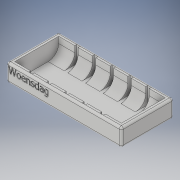
# Autodesk Inventor part: Woendag
Saved by Autodesk Inventor 2019 (Build 230136000, 136)
## iProperties
Created: 2020-10-20
Part Number: Woendag
Material: Generic
Document SubType Name: Modeling
Designer: daanswinters
Density: 1 g/cm^3
Appearance: Default
Author: daanswinters
Autodesk Inventor part; units mm, degrees
ref_plane "YZ Plane" through (0, 0, 0) normal (1, 0, 0) x (0, 1, 0)
ref_plane "XZ Plane" through (0, 0, 0) normal (0, 1, 0) x (-1, 0, 0)
ref_plane "XY Plane" through (0, 0, 0) normal (0, 0, 1) x (1, 0, 0)
sketch "Sketch1" plane through (0, 0, 0) normal (0, 0, 1) x (1, 0, 0)
  line L0 (55, -8.5) -> (-55, -8.5)
  line L1 (-55, -8.5) -> (-55, 8.5)
  line L2 (-55, 8.5) -> (55, 8.5)
  line L3 (55, 8.5) -> (55, -8.5)
  line L4 (55, -8.5) -> (-55, 8.5) construction
  line L5 (-55, -8.5) -> (55, 8.5) construction
  point P0 (0, 0)
  dimension "d0" = 110
  dimension "d1" = 17
  constraints: 12 end point, 2 midpoint, 2 parallel, 1 horizontal, 1 perpendicular
  measures "d0" distance of L1.end L2.end
  measures "d1" distance of L0.end L1.end
extrude "Extrusion1" add sketch "Sketch1" along normal blind 50
sketch "Sketch2" plane through (-55, 8.5, 0) normal (0, 1, 0) x (1, 0, 0)
  line L0 (0, 0) -> (0, -50) projected
  line L1 (110, -50) -> (0, -50)
  line L2 (0, -50) -> (0, 0)
  line L3 (0, 0) -> (110, 0)
  line L4 (110, 0) -> (110, -50)
  line L5 (110, -50) -> (0, 0) construction
  line L6 (0, -50) -> (110, 0) construction
  line L7 (106, -46) -> (106, -4)
  line L8 (4, -4) -> (4, -46)
  line L9 (56.15, -2) -> (53.85, -2)
  line L10 (53.85, -48) -> (56.15, -48)
  line L11 (56.15, -2) -> (53.85, -48) construction
  line L12 (53.85, -2) -> (56.15, -48) construction
  line L13 (73.15, -2) -> (70.85, -2)
  line L14 (70.85, -48) -> (73.15, -48)
  line L15 (73.15, -2) -> (70.85, -48) construction
  line L16 (70.85, -2) -> (73.15, -48) construction
  line L17 (0, -25) -> (110, -25) construction
  line L18 (87.85, -2) -> (90.15, -2)
  line L19 (90.15, -48) -> (87.85, -48)
  line L20 (87.85, -2) -> (90.15, -48) construction
  line L21 (90.15, -2) -> (87.85, -48) construction
  line L22 (36.85, -2) -> (39.15, -2)
  line L23 (39.15, -48) -> (36.85, -48)
  line L24 (36.85, -2) -> (39.15, -48) construction
  line L25 (39.15, -2) -> (36.85, -48) construction
  line L26 (19.85, -2) -> (22.15, -2)
  line L27 (22.15, -48) -> (19.85, -48)
  line L28 (19.85, -2) -> (22.15, -48) construction
  line L29 (22.15, -2) -> (19.85, -48) construction
  line L30 (90.15, -2) -> (90.15, -4)
  line L31 (90.15, -46) -> (90.15, -48)
  line L32 (87.85, -48) -> (87.85, -46)
  line L33 (87.85, -4) -> (87.85, -2)
  line L34 (73.15, -48) -> (73.15, -46)
  line L35 (73.15, -4) -> (73.15, -2)
  line L36 (70.85, -2) -> (70.85, -4)
  line L37 (70.85, -46) -> (70.85, -48)
  line L38 (56.15, -4) -> (56.15, -2)
  line L39 (53.85, -2) -> (53.85, -4)
  line L40 (53.85, -46) -> (53.85, -48)
  line L41 (56.15, -48) -> (56.15, -46)
  line L42 (39.15, -2) -> (39.15, -4)
  line L43 (39.15, -46) -> (39.15, -48)
  line L44 (36.85, -48) -> (36.85, -46)
  line L45 (36.85, -4) -> (36.85, -2)
  line L46 (22.15, -2) -> (22.15, -4)
  line L47 (19.85, -48) -> (19.85, -46)
  line L48 (19.85, -4) -> (19.85, -2)
  line L49 (22.15, -46) -> (22.15, -48)
  line L50 (4, -46) -> (19.95, -46)
  line L51 (22.05, -46) -> (36.95, -46)
  line L52 (39.05, -46) -> (53.95, -46)
  line L53 (56.05, -46) -> (70.95, -46)
  line L54 (73.05, -46) -> (87.95, -46)
  line L55 (90.05, -46) -> (106, -46)
  line L56 (106, -4) -> (90.05, -4)
  line L57 (87.95, -4) -> (73.05, -4)
  line L58 (70.95, -4) -> (56.05, -4)
  line L59 (53.95, -4) -> (39.05, -4)
  line L60 (36.95, -4) -> (22.05, -4)
  line L61 (19.95, -4) -> (4, -4)
  point P0 (55, 0)
  point P1 (55, -25)
  point P2 (72, -25)
  point P3 (89, -25)
  point P4 (38, -25)
  point P5 (21, -25)
  dimension "d4" = 65.556
  dimension "d5" = 110
  dimension "d7" = 2.3
  dimension "d8" = 46
  dimension "d9" = 2.3
  dimension "d10" = 46
  dimension "d11" = 0
  dimension "d12" = 2.3
  dimension "d13" = 46
  dimension "d14" = 2.3
  dimension "d15" = 46
  dimension "d16" = 2.3
  dimension "d17" = 46
  dimension "d18" = 17
  dimension "d19" = 17
  dimension "d20" = 17
  dimension "d21" = 17
  dimension "d22" = 2.862
  dimension "d23" = 2.862
  dimension "d24" = 106
  dimension "d25" = 4
  dimension "d26" = 42
  dimension "d27" = 2
  dimension "d28" = 0
  dimension "d29" = 42
  dimension "d30" = 0
  dimension "d31" = 42
  dimension "d32" = 0
  dimension "d33" = 42
  dimension "d34" = 0
  dimension "d35" = 42
  dimension "d36" = 0
  dimension "d37" = 42
  constraints: 122 end point, 73 parallel, 43 point on line, 17 perpendicular, 14 midpoint, 6 horizontal
  measures "d4" angle of L5 L0
  measures "d5" distance between parallel lines of L4 L0
  measures "d7" distance of L10.end L10.start
  measures "d8" distance of L10.start L9.end
  measures "d9" distance of L14.end L14.start
  measures "d10" distance of L14.start L13.end
  measures "d11" distance from line of L17 point (72, -25)
  measures "d12" distance of L19.start L19.end
  measures "d13" distance of L18.end L19.start
  measures "d14" distance of L23.start L23.end
  measures "d15" distance of L22.end L23.start
  measures "d16" distance of L27.start L27.end
  measures "d17" distance of L26.end L27.start
  measures "d18" distance of point (72, -25) point (55, -25)
  measures "d19" distance of point (89, -25) point (72, -25)
  measures "d20" distance of point (38, -25) point (55, -25)
  measures "d21" distance of point (21, -25) point (38, -25)
  measures "d22" angle of L0 L20
  measures "d23" angle of L0 L21
  measures "d24" distance between parallel lines of L7 L0
  measures "d25" distance between parallel lines of L8 L0
  measures "d26" distance between parallel lines of L56 L55
  measures "d27" distance between parallel lines of L56 L18
  measures "d28" distance between parallel lines of L56 L57
  measures "d29" distance between parallel lines of L56 L54
  measures "d30" distance between parallel lines of L56 L58
  measures "d31" distance between parallel lines of L56 L53
  measures "d32" distance between parallel lines of L56 L59
  measures "d33" distance between parallel lines of L56 L52
  measures "d34" distance between parallel lines of L56 L60
  measures "d35" distance between parallel lines of L56 L51
  measures "d36" distance between parallel lines of L56 L61
  measures "d37" distance between parallel lines of L56 L50
extrude "Extrusion2" cut sketch "Sketch2" against normal blind 16 contours L55 L31 L19 L32 L54 L34 L14 L37 L53 L41 L10 L40 L52 L43 L23 L44 L51 L49 L27 L47 L50 L8 L61 L48 L26 L46 L60 L45 L22 L42 L59 L39 L9 L38 L58 L36 L13 L35 L57 L33 L18 L30 L56 L7
fillet "Fillet1" radius 2 12 edges at (-55, 0, 50) (-55, 0, 0) (55, 0, 50) (55, 0, 0) (0, 8.5, 50) (-55, 8.5, 25) (0, 8.5, 0) (55, 8.5, 25) (55, -8.5, 25) (0, -8.5, 50) (-55, -8.5, 25) (0, -8.5, 0)
fillet "Fillet2" radius 10 6 edges at (-43.075, -7.5, 4) (-25.5, -7.5, 4) (-8.5, -7.5, 4) (8.5, -7.5, 4) (25.5, -7.5, 4) (43.075, -7.5, 4)
sketch "Sketch3" plane through (35.15, 8.5, 4) normal (0, 1, 0) x (1, 0, 0)
  line L0 (-70.3, -44) -> (-70.3, -42) projected
  line L1 (-51, 2) -> (-53.3, 2)
  line L2 (-34, 2) -> (-34, 0) projected
  line L3 (-36.3, -44) -> (-36.3, -42) projected
  line L4 (-19.3, -44) -> (-19.3, -42) projected
  line L5 (-2.3, -44) -> (-2.3, -42) projected
  line L6 (0, 2) -> (0, 0) projected
  line L7 (-19.8, 2) -> (-16.5, 2)
  line L8 (-16.5, 2) -> (-16.5, -44)
  line L9 (-16.5, -44) -> (-19.8, -44)
  line L10 (-19.8, -44) -> (-19.8, 2)
  line L11 (-19.8, 2) -> (-16.5, -44) construction
  line L12 (-16.5, 2) -> (-19.8, -44) construction
  line L13 (-2.8, -44) -> (0.5, -44)
  line L14 (0.5, -44) -> (0.5, 2)
  line L15 (0.5, 2) -> (-2.8, 2)
  line L16 (-2.8, 2) -> (-2.8, -44)
  line L17 (-2.8, -44) -> (0.5, 2) construction
  line L18 (0.5, -44) -> (-2.8, 2) construction
  line L19 (-36.8, -44) -> (-33.5, -44)
  line L20 (-33.5, -44) -> (-33.5, 2)
  line L21 (-33.5, 2) -> (-36.8, 2)
  line L22 (-36.8, 2) -> (-36.8, -44)
  line L23 (-36.8, -44) -> (-33.5, 2) construction
  line L24 (-33.5, -44) -> (-36.8, 2) construction
  line L25 (-51, 2) -> (-36.3, 2) projected
  line L26 (-53.8, -44) -> (-50.5, -44)
  line L27 (-50.5, -44) -> (-50.5, 2)
  line L28 (-50.5, 2) -> (-53.8, 2)
  line L29 (-53.8, 2) -> (-53.8, -44)
  line L30 (-53.8, -44) -> (-50.5, 2) construction
  line L31 (-50.5, -44) -> (-53.8, 2) construction
  line L32 (-53.3, -44) -> (-68, -44) projected
  line L33 (-70.8, 2) -> (-67.5, 2)
  line L34 (-67.5, 2) -> (-67.5, -44)
  line L35 (-67.5, -44) -> (-70.8, -44)
  line L36 (-70.8, -44) -> (-70.8, 2)
  line L37 (-70.8, 2) -> (-67.5, -44) construction
  line L38 (-67.5, 2) -> (-70.8, -44) construction
  point P0 (-35.15, 4)
  point P1 (-68, 2)
  point P2 (-17, 2)
  point P3 (-18.15, -21)
  point P4 (-1.15, -21)
  point P5 (-35.15, -21)
  point P6 (-52.15, -21)
  point P7 (-69.15, -21)
  dimension "d42" = 3.3
  dimension "d43" = 46
  dimension "d44" = 3.3
  dimension "d45" = 3.3
  dimension "d46" = 3.3
  dimension "d47" = 3.3
  dimension "d48" = 90
  dimension "d49" = 0.5
  dimension "d50" = 16.5
  dimension "d51" = 33.5
  dimension "d52" = 50.5
  dimension "d53" = 67.5
  dimension "d54" = 46
  dimension "d55" = 0
  dimension "d56" = 53.3
  constraints: 62 end point, 14 parallel, 10 midpoint, 5 horizontal, 5 perpendicular, 3 point on line
  measures "d42" distance of L8.end L9.end
  measures "d43" distance of L7.end L8.end
  measures "d44" distance of L15.end L14.end
  measures "d45" distance of L21.end L20.end
  measures "d46" distance of L28.end L27.end
  measures "d47" distance of L34.end L35.end
  measures "d48" angle of L6 L1
  measures "d49" distance between parallel lines of L6 L14
  measures "d50" distance between parallel lines of L6 L8
  measures "d51" distance between parallel lines of L6 L20
  measures "d52" distance between parallel lines of L6 L27
  measures "d53" distance between parallel lines of L6 L34
  measures "d54" distance between parallel lines of L25 L9
  measures "d55" distance between parallel lines of L15 L25
  measures "d56" distance from line of L1.end L6
extrude "Extrusion3" cut sketch "Sketch3" against normal blind 16
sketch "Sketch4" plane through (0, 0, 50) normal (0, 0, 1) x (1, 0, 0)
  line L0 (-52.9749, 6.5012) -> (53.0345, 6.5012) construction
  line L1 (53.0345, 6.5012) -> (53.0345, -6.5247) construction
  line L2 (53.0345, -6.5247) -> (-52.9749, -6.5247) construction
  line L3 (-52.9749, -6.5247) -> (-52.9749, 6.5012) construction
  line L4 (-45.5205, 6.2294) -> (-47.0529, 0.1294)
  line L5 (-47.0529, 0.1294) -> (-47.9624, 0.1294)
  line L6 (-47.9624, 0.1294) -> (-49.2032, 5.1913)
  line L7 (-49.2032, 5.1913) -> (-50.4094, 0.1294)
  line L8 (-50.4094, 0.1294) -> (-51.309, 0.1294)
  line L9 (-51.309, 0.1294) -> (-52.8662, 6.2294)
  line L10 (-52.8662, 6.2294) -> (-52.0308, 6.2294)
  line L11 (-52.0308, 6.2294) -> (-50.8048, 1.1724)
  line L12 (-50.8048, 1.1724) -> (-49.5888, 6.2294)
  line L13 (-49.5888, 6.2294) -> (-48.7633, 6.2294)
  line L14 (-48.7633, 6.2294) -> (-47.5373, 1.1131)
  line L15 (-47.5373, 1.1131) -> (-46.3163, 6.2294)
  line L16 (-46.3163, 6.2294) -> (-45.5205, 6.2294)
  spline S0 degree 2 poles (-41.0913, 2.4181) (-41.0913, 1.2614) (-42.2035, 0.0008) (-43.1329, 0.0008) knots 0 0 0 1 2 2 2
  spline S1 degree 2 poles (-43.1329, 0.0008) (-44.0869, 0.0008) (-45.1794, 1.3009) (-45.1794, 2.4181) knots 0 0 0 1 2 2 2
  spline S2 degree 2 poles (-45.1794, 2.4181) (-45.1794, 3.5649) (-44.0523, 4.8354) (-43.1329, 4.8354) knots 0 0 0 1 2 2 2
  spline S3 degree 2 poles (-43.1329, 4.8354) (-42.2035, 4.8354) (-41.0913, 3.5699) (-41.0913, 2.4181) knots 0 0 0 1 2 2 2
  spline S4 degree 2 poles (-41.8872, 2.4181) (-41.8872, 3.3079) (-42.5347, 4.173) (-43.1329, 4.173) knots 0 0 0 1 2 2 2
  spline S5 degree 2 poles (-43.1329, 4.173) (-43.731, 4.173) (-44.3835, 3.3079) (-44.3835, 2.4181) knots 0 0 0 1 2 2 2
  spline S6 degree 2 poles (-44.3835, 2.4181) (-44.3835, 1.553) (-43.731, 0.6632) (-43.1329, 0.6632) knots 0 0 0 1 2 2 2
  spline S7 degree 2 poles (-43.1329, 0.6632) (-42.5397, 0.6632) (-41.8872, 1.5382) (-41.8872, 2.4181) knots 0 0 0 1 2 2 2
  spline S8 degree 2 poles (-38.3132, 0.0256) (-39.4106, 0.0256) (-40.6167, 1.2564) (-40.6167, 2.3934) knots 0 0 0 1 2 2 2
  spline S9 degree 2 poles (-40.6167, 2.3934) (-40.6167, 3.5106) (-39.4452, 4.8354) (-38.501, 4.8354) knots 0 0 0 1 2 2 2
  spline S10 degree 2 poles (-38.501, 4.8354) (-38.0759, 4.8354) (-37.4184, 4.5882) (-37.1762, 4.3262) knots 0 0 0 1 2 2 2
  spline S11 degree 2 poles (-37.1762, 4.3262) (-36.9291, 4.0642) (-36.6671, 3.3079) (-36.6671, 2.7592) knots 0 0 0 1 2 2 2
  line L17 (-36.6671, 2.7592) -> (-36.6671, 2.339)
  line L18 (-36.6671, 2.339) -> (-39.8357, 2.339)
  spline S12 degree 2 poles (-39.8357, 2.339) (-39.8357, 1.5431) (-39.0349, 0.6978) (-38.3231, 0.6978) knots 0 0 0 1 2 2 2
  spline S13 degree 2 poles (-38.3231, 0.6978) (-38.071, 0.6978) (-37.5816, 0.8115) (-37.3838, 0.9005) knots 0 0 0 1 2 2 2
  spline S14 degree 2 poles (-37.3838, 0.9005) (-37.1762, 0.9994) (-36.8895, 1.1724) (-36.7956, 1.2515) knots 0 0 0 1 2 2 2
  line L19 (-36.7956, 1.2515) -> (-36.7511, 1.2515)
  line L20 (-36.7511, 1.2515) -> (-36.7511, 0.4111)
  spline S15 degree 2 poles (-36.7511, 0.4111) (-36.8846, 0.3568) (-37.2899, 0.1986) (-37.4481, 0.1541) knots 0 0 0 1 2 2 2
  spline S16 degree 2 poles (-37.4481, 0.1541) (-37.6706, 0.0898) (-38.0364, 0.0256) (-38.3132, 0.0256) knots 0 0 0 1 2 2 2
  spline S17 degree 2 poles (-37.4184, 2.9273) (-37.4283, 3.2387) (-37.5569, 3.6935) (-37.6804, 3.8467) knots 0 0 0 1 2 2 2
  spline S18 degree 2 poles (-37.6804, 3.8467) (-37.8139, 4.0197) (-38.2341, 4.2026) (-38.5455, 4.2026) knots 0 0 0 1 2 2 2
  spline S19 degree 2 poles (-38.5455, 4.2026) (-38.852, 4.2026) (-39.2821, 4.0197) (-39.46, 3.8418) knots 0 0 0 1 2 2 2
  spline S20 degree 2 poles (-39.46, 3.8418) (-39.633, 3.6589) (-39.811, 3.2189) (-39.8357, 2.9273) knots 0 0 0 1 2 2 2
  line L21 (-39.8357, 2.9273) -> (-37.4184, 2.9273)
  line L22 (-32.2923, 0.1294) -> (-33.0634, 0.1294)
  line L23 (-33.0634, 0.1294) -> (-33.0634, 2.7394)
  spline S21 degree 2 poles (-33.0634, 2.7394) (-33.0634, 3.0558) (-33.1227, 3.5995) (-33.2117, 3.7627) knots 0 0 0 1 2 2 2
  spline S22 degree 2 poles (-33.2117, 3.7627) (-33.3056, 3.9357) (-33.6418, 4.1038) (-33.9285, 4.1038) knots 0 0 0 1 2 2 2
  spline S23 degree 2 poles (-33.9285, 4.1038) (-34.2152, 4.1038) (-34.8232, 3.7973) (-35.1149, 3.5501) knots 0 0 0 1 2 2 2
  line L24 (-35.1149, 3.5501) -> (-35.1149, 0.1294)
  line L25 (-35.1149, 0.1294) -> (-35.886, 0.1294)
  line L26 (-35.886, 0.1294) -> (-35.886, 4.7068)
  line L27 (-35.886, 4.7068) -> (-35.1149, 4.7068)
  line L28 (-35.1149, 4.7068) -> (-35.1149, 4.1977)
  spline S24 degree 2 poles (-35.1149, 4.1977) (-34.7688, 4.5091) (-34.1015, 4.8354) (-33.7258, 4.8354) knots 0 0 0 1 2 2 2
  spline S25 degree 2 poles (-33.7258, 4.8354) (-33.0535, 4.8354) (-32.2923, 3.9456) (-32.2923, 3.1003) knots 0 0 0 1 2 2 2
  line L29 (-32.2923, 3.1003) -> (-32.2923, 0.1294)
  spline S26 degree 2 poles (-29.9739, 0.0206) (-30.4336, 0.0206) (-31.2295, 0.2678) (-31.4915, 0.4062) knots 0 0 0 1 2 2 2
  line L30 (-31.4915, 0.4062) -> (-31.4915, 1.2713)
  line L31 (-31.4915, 1.2713) -> (-31.4519, 1.2713)
  spline S27 degree 2 poles (-31.4519, 1.2713) (-31.353, 1.1922) (-31.0861, 1.0043) (-30.8637, 0.9005) knots 0 0 0 1 2 2 2
  spline S28 degree 2 poles (-30.8637, 0.9005) (-30.6709, 0.8066) (-30.1963, 0.6682) (-29.9442, 0.6682) knots 0 0 0 1 2 2 2
  spline S29 degree 2 poles (-29.9442, 0.6682) (-29.7613, 0.6682) (-29.3411, 0.7522) (-29.2423, 0.8214) knots 0 0 0 1 2 2 2
  spline S30 degree 2 poles (-29.2423, 0.8214) (-29.0989, 0.9153) (-28.9704, 1.1279) (-28.9704, 1.3454) knots 0 0 0 1 2 2 2
  spline S31 degree 2 poles (-28.9704, 1.3454) (-28.9704, 1.6173) (-29.267, 1.8991) (-29.6476, 1.993) knots 0 0 0 1 2 2 2
  spline S32 degree 2 poles (-29.6476, 1.993) (-29.7959, 2.0276) (-30.2705, 2.1265) (-30.4731, 2.1808) knots 0 0 0 1 2 2 2
  spline S33 degree 2 poles (-30.4731, 2.1808) (-30.9971, 2.3341) (-31.4717, 2.9668) (-31.4717, 3.4166) knots 0 0 0 1 2 2 2
  spline S34 degree 2 poles (-31.4717, 3.4166) (-31.4717, 4.0395) (-30.5374, 4.8156) (-29.7663, 4.8156) knots 0 0 0 1 2 2 2
  spline S35 degree 2 poles (-29.7663, 4.8156) (-29.3856, 4.8156) (-28.6145, 4.6277) (-28.3525, 4.4844) knots 0 0 0 1 2 2 2
  line L32 (-28.3525, 4.4844) -> (-28.3525, 3.6589)
  line L33 (-28.3525, 3.6589) -> (-28.392, 3.6589)
  spline S36 degree 2 poles (-28.392, 3.6589) (-28.6886, 3.8961) (-29.4103, 4.168) (-29.7811, 4.168) knots 0 0 0 1 2 2 2
  spline S37 degree 2 poles (-29.7811, 4.168) (-30.1617, 4.168) (-30.6857, 3.8467) (-30.6857, 3.5254) knots 0 0 0 1 2 2 2
  spline S38 degree 2 poles (-30.6857, 3.5254) (-30.6857, 3.2337) (-30.3743, 2.952) (-30.0282, 2.863) knots 0 0 0 1 2 2 2
  spline S39 degree 2 poles (-30.0282, 2.863) (-29.8602, 2.8185) (-29.4351, 2.7295) (-29.2027, 2.6752) knots 0 0 0 1 2 2 2
  spline S40 degree 2 poles (-29.2027, 2.6752) (-28.6985, 2.5466) (-28.1844, 1.9584) (-28.1844, 1.4492) knots 0 0 0 1 2 2 2
  spline S41 degree 2 poles (-28.1844, 1.4492) (-28.1844, 1.1526) (-28.4167, 0.6286) (-28.6441, 0.4359) knots 0 0 0 1 2 2 2
  spline S42 degree 2 poles (-28.6441, 0.4359) (-28.8864, 0.2332) (-29.5043, 0.0206) (-29.9739, 0.0206) knots 0 0 0 1 2 2 2
  line L34 (-23.948, 0.1294) -> (-24.7192, 0.1294)
  line L35 (-24.7192, 0.1294) -> (-24.7192, 0.594)
  spline S43 degree 2 poles (-24.7192, 0.594) (-24.8971, 0.4457) (-25.1591, 0.248) (-25.3371, 0.164) knots 0 0 0 1 2 2 2
  spline S44 degree 2 poles (-25.3371, 0.164) (-25.5002, 0.0849) (-25.8512, 0.0008) (-26.0835, 0.0008) knots 0 0 0 1 2 2 2
  spline S45 degree 2 poles (-26.0835, 0.0008) (-26.4592, 0.0008) (-27.0919, 0.3123) (-27.3144, 0.6138) knots 0 0 0 1 2 2 2
  spline S46 degree 2 poles (-27.3144, 0.6138) (-27.5368, 0.9153) (-27.784, 1.8051) (-27.784, 2.3835) knots 0 0 0 1 2 2 2
  spline S47 degree 2 poles (-27.784, 2.3835) (-27.784, 2.9866) (-27.4726, 3.8665) (-27.2007, 4.1977) knots 0 0 0 1 2 2 2
  spline S48 degree 2 poles (-27.2007, 4.1977) (-26.9486, 4.4943) (-26.2417, 4.8354) (-25.8512, 4.8354) knots 0 0 0 1 2 2 2
  spline S49 degree 2 poles (-25.8512, 4.8354) (-25.5101, 4.8354) (-25.0009, 4.6821) (-24.7192, 4.5239) knots 0 0 0 1 2 2 2
  line L36 (-24.7192, 4.5239) -> (-24.7192, 6.5012)
  line L37 (-24.7192, 6.5012) -> (-23.948, 6.5012)
  line L38 (-23.948, 6.5012) -> (-23.948, 0.1294)
  line L39 (-24.7192, 1.2416) -> (-24.7192, 3.8863)
  spline S50 degree 2 poles (-24.7192, 3.8863) (-25.0059, 4.0247) (-25.4607, 4.1285) (-25.7227, 4.1285) knots 0 0 0 1 2 2 2
  spline S51 degree 2 poles (-25.7227, 4.1285) (-26.3158, 4.1285) (-26.9881, 3.2387) (-26.9881, 2.3983) knots 0 0 0 1 2 2 2
  spline S52 degree 2 poles (-26.9881, 2.3983) (-26.9881, 1.5876) (-26.474, 0.7324) (-25.9056, 0.7324) knots 0 0 0 1 2 2 2
  spline S53 degree 2 poles (-25.9056, 0.7324) (-25.604, 0.7324) (-24.9911, 1.0093) (-24.7192, 1.2416) knots 0 0 0 1 2 2 2
  spline S54 degree 2 poles (-20.2801, 0.6138) (-20.374, 0.5446) (-20.6904, 0.2974) (-20.8387, 0.2233) knots 0 0 0 1 2 2 2
  spline S55 degree 2 poles (-20.8387, 0.2233) (-21.0414, 0.1145) (-21.422, 0.0008) (-21.768, 0.0008) knots 0 0 0 1 2 2 2
  spline S56 degree 2 poles (-21.768, 0.0008) (-22.0498, 0.0008) (-22.559, 0.2134) (-22.7517, 0.4062) knots 0 0 0 1 2 2 2
  spline S57 degree 2 poles (-22.7517, 0.4062) (-22.9347, 0.594) (-23.1571, 1.1477) (-23.1571, 1.4542) knots 0 0 0 1 2 2 2
  spline S58 degree 2 poles (-23.1571, 1.4542) (-23.1571, 1.9287) (-22.7567, 2.601) (-22.3217, 2.7938) knots 0 0 0 1 2 2 2
  spline S59 degree 2 poles (-22.3217, 2.7938) (-21.9361, 2.9718) (-20.8881, 3.1052) (-20.2801, 3.1398) knots 0 0 0 1 2 2 2
  line L40 (-20.2801, 3.1398) -> (-20.2801, 3.2881)
  spline S60 degree 2 poles (-20.2801, 3.2881) (-20.2801, 3.5551) (-20.4432, 3.8863) (-20.5915, 3.9802) knots 0 0 0 1 2 2 2
  spline S61 degree 2 poles (-20.5915, 3.9802) (-20.7398, 4.0741) (-21.165, 4.1334) (-21.3923, 4.1334) knots 0 0 0 1 2 2 2
  spline S62 degree 2 poles (-21.3923, 4.1334) (-21.6593, 4.1334) (-22.381, 3.9752) (-22.7419, 3.822) knots 0 0 0 1 2 2 2
  line L41 (-22.7419, 3.822) -> (-22.7864, 3.822)
  line L42 (-22.7864, 3.822) -> (-22.7864, 4.608)
  spline S63 degree 2 poles (-22.7864, 4.608) (-22.5738, 4.6673) (-21.7779, 4.8156) (-21.3874, 4.8156) knots 0 0 0 1 2 2 2
  spline S64 degree 2 poles (-21.3874, 4.8156) (-20.9129, 4.8156) (-20.2653, 4.6673) (-20.0082, 4.4745) knots 0 0 0 1 2 2 2
  spline S65 degree 2 poles (-20.0082, 4.4745) (-19.7561, 4.2867) (-19.509, 3.6885) (-19.509, 3.2585) knots 0 0 0 1 2 2 2
  line L43 (-19.509, 3.2585) -> (-19.509, 0.1294)
  line L44 (-19.509, 0.1294) -> (-20.2801, 0.1294)
  line L45 (-20.2801, 0.1294) -> (-20.2801, 0.6138)
  line L46 (-20.2801, 1.2564) -> (-20.2801, 2.5269)
  spline S66 degree 2 poles (-20.2801, 2.5269) (-20.5569, 2.5021) (-21.3923, 2.4181) (-21.6543, 2.339) knots 0 0 0 1 2 2 2
  spline S67 degree 2 poles (-21.6543, 2.339) (-21.9608, 2.2451) (-22.3612, 1.8546) (-22.3612, 1.5085) knots 0 0 0 1 2 2 2
  spline S68 degree 2 poles (-22.3612, 1.5085) (-22.3612, 1.1131) (-21.9163, 0.7127) (-21.4912, 0.7127) knots 0 0 0 1 2 2 2
  spline S69 degree 2 poles (-21.4912, 0.7127) (-21.1304, 0.7127) (-20.5372, 1.0241) (-20.2801, 1.2564) knots 0 0 0 1 2 2 2
  spline S70 degree 2 poles (-18.2633, -0.6022) (-18.1842, -0.6368) (-17.8826, -0.7456) (-17.6898, -0.7901) knots 0 0 0 1 2 2 2
  spline S71 degree 2 poles (-17.6898, -0.7901) (-17.4773, -0.8445) (-17.1164, -0.9087) (-16.9039, -0.9087) knots 0 0 0 1 2 2 2
  spline S72 degree 2 poles (-16.9039, -0.9087) (-16.5479, -0.9087) (-16.0536, -0.7209) (-15.9152, -0.5528) knots 0 0 0 1 2 2 2
  spline S73 degree 2 poles (-15.9152, -0.5528) (-15.7817, -0.3847) (-15.6779, 0.0552) (-15.6779, 0.337) knots 0 0 0 1 2 2 2
  line L47 (-15.6779, 0.337) -> (-15.6779, 0.7374)
  spline S74 degree 2 poles (-15.6779, 0.7374) (-15.9894, 0.4655) (-16.5875, 0.2085) (-17.0373, 0.2085) knots 0 0 0 1 2 2 2
  spline S75 degree 2 poles (-17.0373, 0.2085) (-17.8184, 0.2085) (-18.7428, 1.3701) (-18.7428, 2.4626) knots 0 0 0 1 2 2 2
  spline S76 degree 2 poles (-18.7428, 2.4626) (-18.7428, 3.0311) (-18.4214, 3.911) (-18.1545, 4.2224) knots 0 0 0 1 2 2 2
  spline S77 degree 2 poles (-18.1545, 4.2224) (-17.8975, 4.5141) (-17.1906, 4.8354) (-16.8149, 4.8354) knots 0 0 0 1 2 2 2
  spline S78 degree 2 poles (-16.8149, 4.8354) (-16.459, 4.8354) (-15.9399, 4.6673) (-15.6779, 4.5141) knots 0 0 0 1 2 2 2
  line L48 (-15.6779, 4.5141) -> (-15.6334, 4.7068)
  line L49 (-15.6334, 4.7068) -> (-14.9068, 4.7068)
  line L50 (-14.9068, 4.7068) -> (-14.9068, 0.6534)
  spline S79 degree 2 poles (-14.9068, 0.6534) (-14.9068, -0.5133) (-15.9201, -1.6008) (-16.9632, -1.6008) knots 0 0 0 1 2 2 2
  spline S80 degree 2 poles (-16.9632, -1.6008) (-17.2993, -1.6008) (-18.0013, -1.492) (-18.3028, -1.403) knots 0 0 0 1 2 2 2
  line L51 (-18.3028, -1.403) -> (-18.3028, -0.6022)
  line L52 (-18.3028, -0.6022) -> (-18.2633, -0.6022)
  line L53 (-15.6779, 1.3701) -> (-15.6779, 3.8863)
  spline S81 degree 2 poles (-15.6779, 3.8863) (-15.9646, 4.0247) (-16.4491, 4.1433) (-16.6913, 4.1433) knots 0 0 0 1 2 2 2
  spline S82 degree 2 poles (-16.6913, 4.1433) (-17.2746, 4.1433) (-17.9469, 3.2832) (-17.9469, 2.4774) knots 0 0 0 1 2 2 2
  spline S83 degree 2 poles (-17.9469, 2.4774) (-17.9469, 1.7162) (-17.4377, 0.9203) (-16.8643, 0.9203) knots 0 0 0 1 2 2 2
  spline S84 degree 2 poles (-16.8643, 0.9203) (-16.5628, 0.9203) (-15.93, 1.1576) (-15.6779, 1.3701) knots 0 0 0 1 2 2 2
  point P0 (0, 0)
  constraints: 2 other
extrude "Extrusion4" cut sketch "Sketch4" against normal blind 0.5
fillet "Fillet3" radius 10 6 edges at (-43.325, -7.5, 46) (-25.5, -7.5, 46) (-8.5, -7.5, 46) (8.5, -7.5, 46) (25.5, -7.5, 46) (43.325, -7.5, 46)
body "Solid1"
